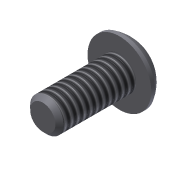
# Autodesk Inventor part: 10-32 x500 button head
Saved by Autodesk Inventor 2013 (Build 170138000, 138)
## iProperties
Created: 2011-07-25
Part Number: 10-32 x500 button head
Material: Steel
Document SubType Name: Modeling
Designer: Dan Niemitalo
Density: 7.85 g/cm^3
Author: Dan Niemitalo
Autodesk Inventor part; units mm, degrees
ref_plane "YZ Plane" through (0, 0, 0) normal (1, 0, 0) x (0, 1, 0)
ref_plane "XZ Plane" through (0, 0, 0) normal (0, 1, 0) x (-1, 0, 0)
ref_plane "XY Plane" through (0, 0, 0) normal (0, 0, 1) x (1, 0, 0)
sketch "Sketch1" plane through (0, 0, 0) normal (0, 0, 1) x (1, 0, 0)
  circle A0 centre (0, 0) radius 2.0828
  dimension "d0" = 4.1656
  constraints: 1 centre point, 1 coincident
  measures "d0" diameter of A0
extrude "Extrusion1" add sketch "Sketch1" along normal blind 9.525
sketch "Sketch2" plane through (0, 0, 0) normal (0, 1, 0) x (-1, 0, 0)
  line L0 (0, 0) -> (0, -2.2098)
  line L1 (0, 0) -> (3.9624, 0)
  line L2 (0, -2.2098) -> (2.032, -2.2098)
  line L3 (3.9624, 0) -> (3.9624, 3.6562) construction
  arc A0 (2.032, -2.2098) -> (3.9624, -0.4599) centre (0.1837, 1.7689) ccw
  line L4 (4.5847, 0.6553) -> (4.5847, -0.2608) construction
  line L5 (3.9624, -0.4599) -> (3.9624, 0)
  dimension "d3" = 2.2098
  dimension "d6" = 2.032
  dimension "d19" = 3.9624
  constraints: 12 end point, 3 point on circle, 2 perpendicular, 2 vertical, 1 centre point, 1 horizontal, 1 parallel
  measures "d3" distance of L0.start L0.end
  measures "d6" distance of L0.end L2.end
  measures "d19" distance between parallel lines of L5 L0
revolve "Revolution1" add sketch "Sketch2" angle 360 about axis through (0, 0, 0) along (0, 0, -1)
sketch "Sketch3" plane through (0, 0, -2.2098) normal (0, 0, -1) x (-1, 0, 0)
  circle A0 centre (0, 0) radius 2.032 projected
  line L0 (-0.6874, 1.1906) -> (0.6874, 1.1906)
  line L1 (0.6874, 1.1906) -> (1.3748, 0)
  line L2 (1.3748, 0) -> (0.6874, -1.1906)
  line L3 (0.6874, -1.1906) -> (-0.6874, -1.1906)
  line L4 (-0.6874, -1.1906) -> (-1.3748, 0)
  line L5 (-1.3748, 0) -> (-0.6874, 1.1906)
  dimension "d8" = 2.3813
  constraints: 12 end point, 1 coincident, 1 horizontal, 13 other
  measures "d8" distance between parallel lines of L3 L0
extrude "Extrusion2" cut sketch "Sketch3" against normal blind 1.5875 contours L0 L1 L2 L3 L4 L5
chamfer "Chamfer1" distance 0.508 angle 45 1 edges at (-2.0828, 0, 9.525)
thread "Thread1" size "8-32 UNC" class "2A" standard "ANSI Unified Screw Threads" full length
body "Solid1"
